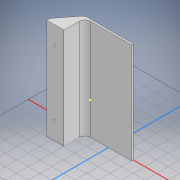
# Autodesk Inventor part: 000.003.002 - Крышка
Saved by Autodesk Inventor 2022 (Build 260153000, 153)
## iProperties
Created: 2023-05-08
Part Number: 000.003.002 - Крышка
Material: Типовые
Document SubType Name: Modeling
Designer: Иван Петров
Density: 1 g/cm^3
Appearance: По умолчанию
Author: Иван Петров
Autodesk Inventor part; units mm, degrees
ref_plane "YZ Plane" through (0, 0, 0) normal (1, 0, 0) x (0, 1, 0)
ref_plane "XZ Plane" through (0, 0, 0) normal (0, 1, 0) x (-1, 0, 0)
ref_plane "XY Plane" through (0, 0, 0) normal (0, 0, 1) x (1, 0, 0)
sketch "Эскиз1" plane through (0, 0, 0) normal (0, 0, 1) x (1, 0, 0)
  line L0 (40, -86.25) -> (-40, -86.25)
  line L1 (-40, -86.25) -> (-40, 86.25)
  line L2 (-40, 86.25) -> (40, 86.25)
  line L3 (40, 86.25) -> (40, -86.25)
  line L4 (40, -86.25) -> (-40, 86.25) construction
  line L5 (-40, -86.25) -> (40, 86.25) construction
  point P0 (0, 0)
  dimension "d0" = 80
  dimension "d1" = 172.5
  constraints: 12 end point, 2 midpoint, 2 parallel, 1 horizontal, 1 perpendicular
  measures "d0" distance of L1.end L2.end
  measures "d1" distance of L0.end L1.end
extrude "Выдавливание1" add sketch "Эскиз1" along normal blind 3
sketch "Эскиз2" plane through (-40, -86.25, 0) normal (-1, 0, 0) x (0, 0, 1)
  line L0 (0, 172.5) -> (39, 172.5)
  line L1 (39, 172.5) -> (39, 0)
  line L2 (39, 0) -> (0, 0)
  line L3 (0, 0) -> (0, 172.5)
  dimension "d4" = 39
  constraints: 8 end point, 2 parallel, 1 horizontal, 1 perpendicular, 1 point on line
  measures "d4" distance between parallel lines of L1 L3
extrude "Выдавливание2" add sketch "Эскиз2" along normal blind 3
sketch "Эскиз3" plane through (-43, -86.25, 0) normal (-1, 0, 0) x (0, 0, 1)
  line L0 (3, 0) -> (39, 0) projected
  line L1 (39, 172.5) -> (3, 172.5) projected
  line L2 (39, 0) -> (34, 0)
  line L3 (34, 0) -> (34, 172.5)
  line L4 (34, 172.5) -> (39, 172.5)
  line L5 (39, 172.5) -> (39, 0)
  point P0 (0, 86.25)
  point P1 (34, 0)
  dimension "d7" = 5
  constraints: 8 end point, 2 parallel, 1 horizontal, 1 perpendicular, 1 point on line
  measures "d7" distance between parallel lines of L5 L3
extrude "Выдавливание3" add sketch "Эскиз3" along normal blind 26.5
sketch "Эскиз4" plane through (-43, -86.25, 34) normal (0, 0, -1) x (-1, 0, 0)
  point P0 (-43, 86.25)
sketch "Эскиз5" plane through (-43, -86.25, 34) normal (0, 0, -1) x (-1, 0, 0)
  circle A0 centre (13, 30.25) radius 1.85 projected
  circle A1 centre (13, 142.25) radius 1.85 projected
  point P0 (-43, 86.25)
extrude "Выдавливание4" cut sketch "Эскиз5" against normal blind 26.5
sketch "Эскиз6" plane through (40, 86.25, 3) normal (0, 1, 0) x (1, 0, 0)
  line L0 (0, 3) -> (-83, 3) projected
  line L1 (-83, -31) -> (-109.5, -31) projected
  line L2 (-83, 3) -> (-109.5, -31)
  line L3 (-83, 3) -> (-83, -31) projected
  line L4 (-83, 3) -> (-83, -31)
  line L5 (-80, 0) -> (-80, -36) projected
  point P0 (-40, 3)
  constraints: 4 end point, 1 parallel
extrude "Выдавливание5" add sketch "Эскиз6" against normal up to surface (172.5 mm away)
ref_plane "РабПлоскость1" through (-69.5, 86.25, 34) normal (0, 0, -1) x (0, -1, 0)
sketch "Эскиз7" plane through (-69.5, 86.25, 34) normal (0, 0, -1) x (0, -1, 0)
  circle A0 centre (142.25, -13.5) radius 1.85 projected
  circle A1 centre (30.25, -13.5) radius 1.85 projected
  circle A2 centre (30.25, -13.5) radius 1.85 projected
  circle A3 centre (30.25, -13.5) radius 5
  circle A4 centre (142.25, -13.5) radius 1.85 projected
  circle A5 centre (142.25, -13.5) radius 5
  point P0 (86.25, -69.5)
  dimension "d15" = 10
  dimension "d16" = 10
  constraints: 2 centre point, 2 coincident
  measures "d15" diameter of A3
  measures "d16" diameter of A5
extrude "Выдавливание6" cut sketch "Эскиз7" along normal blind 36.75 contours A0 | A1 | A3 | A5
fillet "Сопряжение1" radius 10 2 edges at (-40, 0, 3) (-43, 0, 0)
fillet "Сопряжение2" radius 10 1 edges at (-69.5, 0, 34)
equation "\"d16\" = d15"
